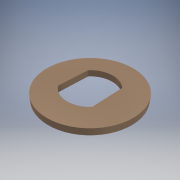
# Autodesk Inventor part: PODKŁADKA M8X6X18
Saved by Autodesk Inventor 2017 SP1 (Build 210196100, 196)
## iProperties
Created: 2021-01-30
Part Number: PODKŁADKA M8X6X18
Material: Stal
Document SubType Name: Modeling
Designer: Napoleon
Density: 7.85 g/cm^3
Appearance: Anodowany - brązowy
Mass: 1.04033 g
Surface Area: 3.36171 cm^2
Volume: 0.132526 cm^3
Author: Napoleon
Autodesk Inventor part; units mm, degrees
ref_plane "YZ Plane" through (0, 0, 0) normal (1, 0, 0) x (0, 1, 0)
ref_plane "XZ Plane" through (0, 0, 0) normal (0, 1, 0) x (-1, 0, 0)
ref_plane "XY Plane" through (0, 0, 0) normal (0, 0, 1) x (1, 0, 0)
sketch "Szkic1" plane through (0, 0, 0) normal (0, 0, 1) x (1, 0, 0)
  circle A0 centre (0, 0) radius 7.475
  line L0 (-3, -2.6458) -> (-3, 2.6458)
  line L1 (3, -2.6458) -> (3, 2.6458)
  arc A1 (-3, -2.6458) -> (3, -2.6458) centre (0, 0) ccw
  arc A2 (3, 2.6458) -> (-3, 2.6458) centre (0, 0) ccw
  constraints: 4 end point, 4 point on circle, 3 centre point, 1 coincident, 1 vertical
extrude "Wyciągnięcie proste1" add sketch "Szkic1" along normal mid plane 1
